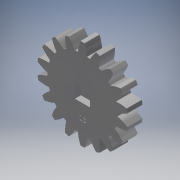
# Autodesk Inventor part: 18_teeth
Saved by Autodesk Inventor 2019 (Build 230136000, 136)
## iProperties
Created: 2020-02-24
Part Number: 18_teeth
Material: Steel
Document SubType Name: Modeling
Designer: Jeff
Categories: <?xml version="1.0" encoding="UTF-16"?> <MemberInstance><Categories><FamilyTemplate><FamilyTemplateParameter ValueType="xs:double" Id="1" ObjectReferenceKey="da_z" ObjectType="kUserParameterObject"/><FamilyTemplateParameter ValueType="xs:double" Id="2" ObjectReferenceKey="da_b" ObjectType="kUserParameterObject"/><FamilyTemplateParameter ValueType="xs:double" Id="3" ObjectReferenceKey="da_beta" ObjectType="kUserParameterObject"/><FamilyTemplateParameter ValueType="xs:double" Id="4" ObjectReferenceKey="da_da" ObjectType="kUserParameterObject"/><FamilyTemplateParameter ValueType="xs:double" Id="5" ObjectReferenceKey="da_aw" ObjectType="kUserParameterObject"/><FamilyTemplateParameter ValueType="xs:string" Id="6" ObjectReferenceKey="EAIAABAAAACIAQAAAAAAAIAAAAAAAAAA" ObjectType="83910656" SubObjectId="SurfaceGeometry"/></FamilyTemplate><ParamToTemplateMap><ParamToTemplate CategoryParameter="//CategoryParameter[@InternalName='046C89C9-8512-4d59-83FE-43B91F4F132A']" TemplateParameter="1"/><ParamToTemplate CategoryParameter="//CategoryParameter[@InternalName='2552DF32-E462-4b46-AEBF-C6C7768E72AC']" TemplateParameter="2"/><ParamToTemplate CategoryParameter="//CategoryParameter[@InternalName='C9EE641D-15FC-4fae-A226-E94C4372FDD7']" TemplateParameter="3"/><ParamToTemplate><ParamToTemplate CategoryParameter="//CategoryParameter[@InternalName='00B6519A-459B-49c7-AD84-2E56D39A5744']" ConstantValue="0.000000"/></ParamToTemplate><ParamToTemplate><ParamToTemplate CategoryParameter="//CategoryParameter[@InternalName='04B31F0E-C7A6-4894-AA32-9629BEFACF47']" ConstantValue="1.000000"/></ParamToTemplate><ParamToTemplate><ParamToTemplate CategoryParameter="//CategoryParameter[@InternalName='43CBEC2E-7847-49e7-A936-2F7889FCB2D9']" ConstantValue="0.250000"/></ParamToTemplate><ParamToTemplate><ParamToTemplate CategoryParameter="//CategoryParameter[@InternalName='B1EFC894-105D-4ebd-86BF-FA20ED196853']" ConstantValue="0.350000"/></ParamToTemplate><ParamToTemplate><ParamToTemplate CategoryParameter="//CategoryParameter[@InternalName='51175063-3D10-4879-93E8-6246FE8B403D']" ConstantValue="2060000000.000000"/></ParamToTemplate><ParamToTemplate><ParamToTemplate CategoryParameter="//CategoryParameter[@InternalName='A3A52E27-4454-46a9-B0BD-C932399B70AF']" ConstantValue="0.300000"/></ParamToTemplate><ParamToTemplate><ParamToTemplate CategoryParameter="//CategoryParameter[@InternalName='91B76062-C214-41d9-B1B9-14D2AB99603D']" ConstantValue="0.300000"/></ParamToTemplate><ParamToTemplate><ParamToTemplate CategoryParameter="//CategoryParameter[@InternalName='374E806E-8B8A-4dda-A9AA-1039D6500AD2']" ConstantValue="3.333333"/></ParamToTemplate><ParamToTemplate><ParamToTemplate CategoryParameter="//CategoryParameter[@InternalName='2D373A89-B862-43d6-8D0B-0CBF12AB9F6C']" ConstantValue="0.349066"/></ParamToTemplate><ParamToTemplate CategoryParameter="//CategoryParameter[@InternalName='37777632-D6A2-4fac-9D53-DB8ACD95C989']" TemplateParameter="4"/><ParamToTemplate CategoryParameter="//CategoryParameter[@InternalName='FD1017F1-B727-4f7e-9707-0F86F1FF9423']" TemplateParameter="5"/><ParamToTemplate><ParamToTemplate CategoryParameter="//CategoryParameter[@InternalName='9E1B4470-B2D3-4ff1-B813-535BB4CDF51A']" ConstantValue="3520000.000000"/></ParamToTemplate><ParamToTemplate><ParamToTemplate CategoryParameter="//CategoryParameter[@InternalName='F8452263-BFF6-458c-9FB1-07C4B99E95CD']" ConstantValue="11400000.000000"/></ParamToTemplate><ParamToTemplate><ParamToTemplate CategoryParameter="//CategoryParameter[@InternalName='3E3BB259-FD49-497f-8171-6EBC954A3479']" ConstantValue="2.000000"/></ParamToTemplate><ParamToTemplate CategoryParameter="//CategoryParameter[@InternalName='27C3BAF2-7550-4e4b-AE2C-0DB134B7D9B7']" TemplateParameter="6"/></ParamToTemplateMap><Category DisplayName="Gear" InternalName="DC85795E-93AB-48d5-8EEE-5A27447B64BD" Mnemonic="Gear"><CategoryParameter DisplayName="z" InternalName="046C89C9-8512-4d59-83FE-43B91F4F132A" Mnemonic="z"/><CategoryParameter DisplayName="b" InternalName="2552DF32-E462-4b46-AEBF-C6C7768E72AC" Mnemonic="b"/><CategoryParameter DisplayName="||b|" InternalName="C9EE641D-15FC-4fae-A226-E94C4372FDD7" Mnemonic="beta"/><CategoryParameter DisplayName="x" InternalName="00B6519A-459B-49c7-AD84-2E56D39A5744" Mnemonic="x"/><CategoryParameter DisplayName="a*" InternalName="04B31F0E-C7A6-4894-AA32-9629BEFACF47" Mnemonic="a"/><CategoryParameter DisplayName="c*" InternalName="43CBEC2E-7847-49e7-A936-2F7889FCB2D9" Mnemonic="c"/><CategoryParameter DisplayName="r|.f|*" InternalName="B1EFC894-105D-4ebd-86BF-FA20ED196853" Mnemonic="rf"/><CategoryParameter DisplayName="E" InternalName="51175063-3D10-4879-93E8-6246FE8B403D" Mnemonic="E"/><CategoryParameter DisplayName="||m|" InternalName="A3A52E27-4454-46a9-B0BD-C932399B70AF" Mnemonic="mi"/><Category DisplayName="SpurGear" InternalName="26C5A22E-A91E-4dfd-A3B3-23CCAFAE1764" Mnemonic="SpurGear"><CategoryParameter DisplayName="m" InternalName="91B76062-C214-41d9-B1B9-14D2AB99603D" Mnemonic="m"/><CategoryParameter DisplayName="P" InternalName="374E806E-8B8A-4dda-A9AA-1039D6500AD2" Mnemonic="PP"/><CategoryParameter DisplayName="||a|" InternalName="2D373A89-B862-43d6-8D0B-0CBF12AB9F6C" Mnemonic="alpha"/><CategoryParameter DisplayName="d|.a|" InternalName="37777632-D6A2-4fac-9D53-DB8ACD95C989" Mnemonic="da"/><CategoryParameter DisplayName="a|.w|" InternalName="FD1017F1-B727-4f7e-9707-0F86F1FF9423" Mnemonic="aw"/><CategoryParameter DisplayName="||s||.Flim|" InternalName="9E1B4470-B2D3-4ff1-B813-535BB4CDF51A" Mnemonic="sFlim"/><CategoryParameter DisplayName="||s||.Hlim|" InternalName="F8452263-BFF6-458c-9FB1-07C4B99E95CD" Mnemonic="sHlim"/><CategoryParameter DisplayName="type" InternalName="3E3BB259-FD49-497f-8171-6EBC954A3479" Mnemonic="type"/><CategoryParameter DisplayName="PitchDiameter" InternalName="27C3BAF2-7550-4e4b-AE2C-0DB134B7D9B7" Mnemonic="IDS_PITCHDIAM"/></Category></Category></Categories></MemberInstance>
Density: 1 g/cm^3
Appearance: Steel
CustomPartVersion: 1
Author: Jeff
Autodesk Inventor part; units mm, degrees
sketch "Sketch1" plane through (0, 0, 0) normal (0, 0, 1) x (1, 0, 0)
  circle A0 centre (0, 0) radius 30
  dimension "d0" = 60
  constraints: 1 centre point
  measures "d0" diameter of A0
extrude "Extrusion1" add sketch "Sketch1" along normal blind 10
ref_plane "Work Plane2" through (0, 0, 5) normal (0, 0, 1) x (1, 0, 0)
sketch "Sketch2" plane through (0, 0, 0) normal (0, 0, -1) x (-1, 0, 0)
  circle A0 centre (0, 0) radius 30 projected
  circle A1 centre (0, 0) radius 27
  dimension "d3" = 54
  constraints: 1 centre point, 1 coincident
  measures "d3" diameter of A1
surface extrude "Pitch Diameter" sketch "Sketch2" against normal through all shown no curves A1
ref_plane "Work Plane8" through (0, 0, 0) normal (0.9848078, 0.1736482, 0) x (0, 0, 1)
ref_plane "Work Plane9" through (0, 0, 0) normal (1, 0, 0) x (0, 1, 0)
spur gear teeth "Spur Gear" teeth 18 pitch diameter 54 tip diameter 60 root diameter 46.5 face width 10 start plane through (0, 0, 0) normal (0, 0, -1) x (-1, 0, 0)
sketch "Sketch3" plane through (0, 0, 10) normal (0, 0, 1) x (1, 0, 0)
  line L0 (-5, 5) -> (5, 5)
  line L1 (5, 5) -> (5, -5)
  line L2 (5, -5) -> (-5, -5)
  line L3 (-5, -5) -> (-5, 5)
  line L4 (-5, -19.0255) -> (-5, -9.0255) construction
  line L5 (-5, -9.0255) -> (5, -9.0255) construction
  line L6 (5, -9.0255) -> (5, -19.0255) construction
  line L7 (5, -19.0255) -> (-5, -19.0255) construction
  arc A0 (-5.0322, -22.6989) -> (-3.0347, -23.0511) centre (0, 0) ccw projected
  line L8 (-3.0347, -23.0511) -> (-3.0347, -5)
  line L9 (-0.3331, -15.5255) -> (-1.7966, -15.5255)
  line L10 (-1.7966, -15.5255) -> (-1.7966, -15.2192)
  line L11 (-1.7966, -15.2192) -> (-1.252, -15.2192)
  line L12 (-1.252, -15.2192) -> (-1.252, -13.2087)
  line L13 (-1.252, -13.2087) -> (-1.7966, -13.2087)
  line L14 (-1.7966, -13.2087) -> (-1.7966, -12.934)
  spline S0 degree 2 poles (-1.7966, -12.934) (-1.4878, -12.934) (-1.1961, -12.7589) (-1.1767, -12.5158) knots 0 0 0 1 2 2 2
  line L15 (-1.1767, -12.5158) -> (-0.8655, -12.5158)
  line L16 (-0.8655, -12.5158) -> (-0.8655, -15.2192)
  line L17 (-0.8655, -15.2192) -> (-0.3331, -15.2192)
  line L18 (-0.3331, -15.2192) -> (-0.3331, -15.5255)
  spline S1 degree 2 poles (1.1256, -15.5936) (0.9019, -15.5936) (0.5348, -15.4599) (0.406, -15.3359) knots 0 0 0 1 2 2 2
  spline S2 degree 2 poles (0.406, -15.3359) (0.2796, -15.2144) (0.1483, -14.8837) (0.1483, -14.6965) knots 0 0 0 1 2 2 2
  spline S3 degree 2 poles (0.1483, -14.6965) (0.1483, -14.4534) (0.4084, -14.045) (0.6564, -13.9234) knots 0 0 0 1 2 2 2
  line L19 (0.6564, -13.9234) -> (0.6564, -13.9113)
  spline S4 degree 2 poles (0.6564, -13.9113) (0.4352, -13.7824) (0.2212, -13.4761) (0.2212, -13.2476) knots 0 0 0 1 2 2 2
  spline S5 degree 2 poles (0.2212, -13.2476) (0.2212, -12.9097) (0.7318, -12.4575) (1.1256, -12.4575) knots 0 0 0 1 2 2 2
  spline S6 degree 2 poles (1.1256, -12.4575) (1.534, -12.4575) (2.0276, -12.8854) (2.0276, -13.2208) knots 0 0 0 1 2 2 2
  spline S7 degree 2 poles (2.0276, -13.2208) (2.0276, -13.4226) (1.7917, -13.8165) (1.5705, -13.9283) knots 0 0 0 1 2 2 2
  line L20 (1.5705, -13.9283) -> (1.5705, -13.9405)
  spline S8 degree 2 poles (1.5705, -13.9405) (1.8331, -14.062) (2.1029, -14.4121) (2.1029, -14.6892) knots 0 0 0 1 2 2 2
  spline S9 degree 2 poles (2.1029, -14.6892) (2.1029, -15.0734) (1.5438, -15.5936) (1.1256, -15.5936) knots 0 0 0 1 2 2 2
  spline S10 degree 2 poles (1.6896, -14.7281) (1.6896, -14.5434) (1.5438, -14.3246) (1.3371, -14.2127) knots 0 0 0 1 2 2 2
  spline S11 degree 2 poles (1.3371, -14.2127) (1.269, -14.1738) (1.0405, -14.0839) (0.8971, -14.0255) knots 0 0 0 1 2 2 2
  spline S12 degree 2 poles (0.8971, -14.0255) (0.7318, -14.1349) (0.5543, -14.4607) (0.5543, -14.6674) knots 0 0 0 1 2 2 2
  spline S13 degree 2 poles (0.5543, -14.6674) (0.5543, -14.9396) (0.8825, -15.2946) (1.1305, -15.2946) knots 0 0 0 1 2 2 2
  spline S14 degree 2 poles (1.1305, -15.2946) (1.3833, -15.2946) (1.6896, -14.9907) (1.6896, -14.7281) knots 0 0 0 1 2 2 2
  spline S15 degree 2 poles (1.6337, -13.2257) (1.6337, -13.0239) (1.3639, -12.7541) (1.1232, -12.7541) knots 0 0 0 1 2 2 2
  spline S16 degree 2 poles (1.1232, -12.7541) (0.9044, -12.7541) (0.6248, -12.9948) (0.6248, -13.2014) knots 0 0 0 1 2 2 2
  spline S17 degree 2 poles (0.6248, -13.2014) (0.6248, -13.3497) (0.7682, -13.5563) (0.9117, -13.639) knots 0 0 0 1 2 2 2
  spline S18 degree 2 poles (0.9117, -13.639) (0.9724, -13.673) (1.2301, -13.7922) (1.3347, -13.8262) knots 0 0 0 1 2 2 2
  spline S19 degree 2 poles (1.3347, -13.8262) (1.5097, -13.6925) (1.6337, -13.408) (1.6337, -13.2257) knots 0 0 0 1 2 2 2
  point P0 (0, 5)
  point P1 (5, 0)
  point P2 (0, -9.0255)
  point P3 (-5, -14.0255)
  point P4 (-3.0347, -14.0255)
  dimension "d49" = 10
  dimension "d50" = 10
  dimension "d56" = 10
  dimension "d57" = 10
  constraints: 10 end point, 5 midpoint, 2 horizontal, 2 horizontal alignment, 2 parallel, 2 perpendicular, 1 point on line, 1 vertical alignment, 2 other
  measures "d49" distance of L1.end L2.end
  measures "d50" distance of L0.end L1.end
  measures "d56" distance between parallel lines of L6 L4
  measures "d57" distance between parallel lines of L5 L7
extrude "Extrusion2" cut sketch "Sketch3" against normal blind 4
sketch "Sketch4" plane through (0, 0, 0) normal (0, 0, -1) x (-1, 0, 0)
  circle A0 centre (0, 0) radius 7.5
  dimension "d53" = 15
  constraints: 1 centre point, 1 coincident
  measures "d53" diameter of A0
extrude "Extrusion3" cut sketch "Sketch4" against normal blind 4
equation "\"d0\" = da_da"
equation "\"d1\" = da_b"
equation "\"d3\" = da_dw"
equation "\"d16\" = da_aw"
equation "\"d43\" = da_aw"
equation "\"d46\" = da_aw"
equation "\"da_da\" = 60"
equation "\"da_b\" = 10"
equation "\"da_dw\" = 54"
equation "\"da_aw\" = 42"
body "Solid1"
body "Srf1"
